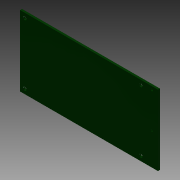
# Autodesk Inventor part: BetaBoard01
Saved by Autodesk Inventor 2013 (Build 170138000, 138)
## iProperties
Created: 2014-04-13
Part Number: BetaBoard01
Material: PCB(1)
Document SubType Name: Modeling
Designer: spichelh
Density: 1 g/cm^3
Author: spichelh
Autodesk Inventor part; units mm, degrees
ref_plane "YZ Plane" through (0, 0, 0) normal (1, 0, 0) x (0, 1, 0)
ref_plane "XZ Plane" through (0, 0, 0) normal (0, 1, 0) x (-1, 0, 0)
ref_plane "XY Plane" through (0, 0, 0) normal (0, 0, 1) x (1, 0, 0)
sketch "Sketch1" plane through (0, 0, 0) normal (0, 0, 1) x (1, 0, 0)
  line L0 (-55.88, -28.575) -> (55.88, -28.575)
  line L1 (55.88, -28.575) -> (55.88, 28.575)
  line L2 (55.88, 28.575) -> (-55.88, 28.575)
  line L3 (-55.88, 28.575) -> (-55.88, -28.575)
  line L4 (-55.88, -28.575) -> (55.88, 28.575) construction
  line L5 (55.88, -28.575) -> (-55.88, 28.575) construction
  circle A0 centre (-52.07, 24.765) radius 1.4
  line L6 (-55.88, 0) -> (55.88, 0) construction
  line L7 (0, 28.575) -> (0, -28.575) construction
  circle A1 centre (-52.07, -24.765) radius 1.4
  circle A2 centre (-31.75, 24.765) radius 1.4
  circle A3 centre (31.75, 24.765) radius 1.4
  circle A4 centre (-31.75, -24.765) radius 1.4
  circle A5 centre (31.75, -24.765) radius 1.4
  circle A6 centre (50.8, 25.865) radius 0.99
  circle A7 centre (41.91, 24.765) radius 1.4
  circle A8 centre (41.91, -24.765) radius 1.4
  circle A9 centre (50.8, -2.71) radius 0.8
  point P0 (0, 0)
  dimension "d2" = 111.76
  dimension "d4" = 57.15
  dimension "d5" = 49.53
  dimension "d6" = 2.8
  dimension "d8" = 2.8
  dimension "d10" = 49.53
  dimension "d21" = 3.81
  dimension "d22" = 3.81
  dimension "d23" = 3.81
  dimension "d28" = 3.81
  dimension "d30" = 63.5
  dimension "d35" = 1.98
  dimension "d36" = 5.08
  dimension "d37" = 2.71
  dimension "d38" = 2.8
  dimension "d39" = 3.81
  dimension "d40" = 13.97
  dimension "d41" = 63.5
  dimension "d42" = 1.6
  dimension "d43" = 5.08
  dimension "d44" = 2.71
  constraints: 16 end point, 10 centre point, 6 midpoint, 5 symmetric about line, 2 parallel, 1 horizontal, 1 perpendicular, 5 other
  measures "d2" distance of L1.end L2.end
  measures "d4" distance of L0.end L1.end
  measures "d5" distance of A1.centre A0.centre
  measures "d6" diameter of A1
  measures "d8" diameter of A2
  measures "d10" distance of A4.centre A2.centre
  measures "d21" distance from line of L0 A4.centre
  measures "d22" distance from line of L3 A0.centre
  measures "d23" distance from line of L2 A0.centre
  measures "d28" distance from line of L0 A5.centre
  measures "d30" distance of A3.centre A2.centre
  measures "d35" diameter of A6
  measures "d36" distance from line of L1 A6.centre
  measures "d37" distance from line of L2 A6.centre
  measures "d38" diameter of A7
  measures "d39" distance from line of L2 A7.centre
  measures "d40" distance from line of L1 A7.centre
  measures "d41" distance of A5.centre A4.centre
  measures "d42" diameter of A9
  measures "d43" distance from line of L1 A9.centre
  measures "d44" vertical distance of A9.centre L6.end
extrude "Extrusion1" add sketch "Sketch1" along normal blind 1.6 contours L3 L2 L1 L0 | A2 | A3 | A4 | A5
sketch "Sketch3" plane through (0, 0, 1.6) normal (0, 0, 1) x (1, 0, 0)
  circle A0 centre (26.67, -24.765) radius 1.4 projected
  circle A1 centre (-26.67, -24.765) radius 1.4 projected
  line L0 (55.88, 28.575) -> (-55.88, 28.575) projected
  line L1 (-21.67, -25.765) -> (21.67, -25.765)
  line L2 (21.67, -25.765) -> (21.67, 30.575)
  line L3 (21.67, 30.575) -> (-21.67, 30.575)
  line L4 (-21.67, 30.575) -> (-21.67, -25.765)
  line L5 (55.88, -28.575) -> (55.88, 28.575) projected
  line L6 (-55.88, 28.575) -> (-55.88, -28.575) projected
  point P0 (0, 0)
  dimension "d15" = 2
  dimension "d16" = 5
  dimension "d17" = 5
  dimension "d18" = 1
  dimension "d33" = 34.21
  dimension "d34" = 34.21
  constraints: 8 end point, 2 parallel, 1 horizontal, 1 perpendicular
  measures "d15" distance between parallel lines of L0 L3
  measures "d16" distance from line of A0.centre L2
  measures "d17" distance from line of A1.centre L4
  measures "d18" distance from line of A0.centre L1
  measures "d33" distance between parallel lines of L6 L4
  measures "d34" distance between parallel lines of L5 L2
extrude "Extrusion3" [suppressed]
body "Solid1"
